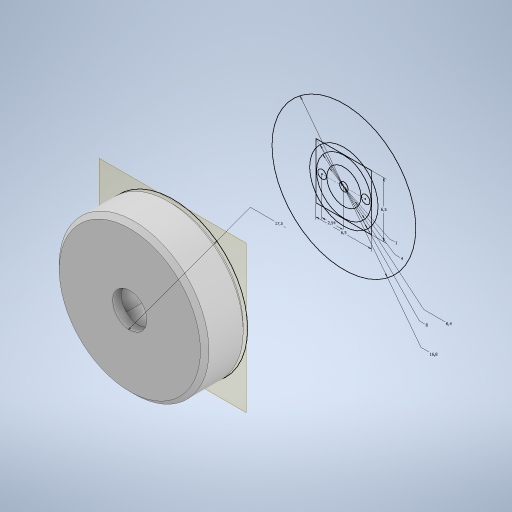
# Autodesk Inventor part: ATT_BUTN
Saved by Autodesk Inventor 2024 (Build 280153000, 153)
## iProperties
Created: 2024-11-27
Part Number: ATT_BUTN
Material: Типовые
Document SubType Name: Modeling
Designer: fm
Density: 1 g/cm^3
Appearance: По умолчанию
Author: fm
Autodesk Inventor part; units mm, degrees
ref_plane "YZ Plane" through (0, 0, 0) normal (1, 0, 0) x (0, 1, 0)
ref_plane "XZ Plane" through (0, 0, 0) normal (0, 1, 0) x (-1, 0, 0)
ref_plane "XY Plane" through (0, 0, 0) normal (0, 0, 1) x (1, 0, 0)
sketch "Эскиз1" plane through (0, 0, 0) normal (0, 0, 1) x (1, 0, 0)
  circle A0 centre (0, 0) radius 3.2
  circle A1 centre (0, 0) radius 8.4
  circle A2 centre (0, 0) radius 0.5
  circle A3 centre (2.54, 0) radius 0.5
  circle A4 centre (-2.54, 0) radius 0.5
  circle A5 centre (0, 0) radius 4
  line L0 (-2.54, 0) -> (2.54, 0) construction
  circle A6 centre (0, 0) radius 2
  line L1 (-3.25, 3.25) -> (3.25, 3.25)
  line L2 (3.25, 3.25) -> (3.25, -3.25)
  line L3 (3.25, -3.25) -> (-3.25, -3.25)
  line L4 (-3.25, -3.25) -> (-3.25, 3.25)
  line L5 (-3.25, 3.25) -> (3.25, -3.25) construction
  point P0 (3.1401, 0.2498)
  point P1 (-3.1401, 0.2498)
  point P2 (-3.1401, -0.2498)
  point P3 (3.1401, -0.2498)
  dimension "d0" = 6.4
  dimension "d1" = 16.8
  dimension "d2" = 1
  dimension "d7" = 8
  dimension "d9" = 2.54
  dimension "d10" = 4
  dimension "d33" = 6.5
  dimension "d34" = 6.5
  constraints: 12 end point, 8 coincident, 7 centre point, 2 equal radius, 2 horizontal, 2 midpoint, 2 parallel, 1 perpendicular
  measures "d0" diameter of A0
  measures "d1" diameter of A1
  measures "d2" diameter of A2
  measures "d7" diameter of A5
  measures "d9" distance of point (0, 0) L0.start
  measures "d10" diameter of A6
  measures "d33" distance of L2.end L3.end
  measures "d34" distance of L1.end L2.end
extrude "Выдавливание1" add sketch "Эскиз1" against normal blind 2 contours A0 | A1 | A2 | A5 L2 | L2 A5 L3 L4 L1 | A5 L1 L2 | L2 L3 A5 | L1 A5 | A5 L3 | A5 L4 L1 | L3 L4 A5 | L4 A5 | A6
chamfer "Фаска1" distance 0.5 angle 45 1 edges at (-8.4, 0, -2)
ref_plane "РабПлоскость1" through (0, 0, 20) normal (0, 0, 1) x (1, 0, 0)
sketch "Эскиз2" plane through (0, 0, 20) normal (0, 0, 1) x (1, 0, 0)
  circle A0 centre (0, 0) radius 8.75
  dimension "d23" = 17.5
  constraints: 1 centre point, 1 coincident
  measures "d23" diameter of A0
extrude "Выдавливание5" add sketch "Эскиз2" along normal blind 5 separate body
extrude "Выдавливание6" cut sketch "Эскиз1" along normal up to surface (5 mm away) from surface at 20 contours A2 | A6 bodies 2
extrude "Выдавливание7" cut sketch "Эскиз1" along normal blind 4 from surface at 20 contours A0 | A2 | A3 | A4 | L2 A5 L3 L4 L1 | A5 L1 L2 | L2 L3 A5 | A5 L4 L1 | L3 L4 A5 | A6 bodies 2
chamfer "Фаска2" distance 0.5 angle 45 2 edges at (-8.75, 0, 20) (-8.75, 0, 25)
